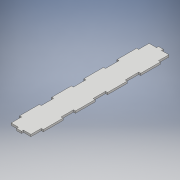
# Autodesk Inventor part: F3
Saved by Autodesk Inventor 2018 (Build 220112000, 112)
## iProperties
Created: 2018-03-06
Part Number: F3
Material: Generic
Document SubType Name: Modeling
Designer: isai
Density: 1 g/cm^3
Appearance: Default
Author: isai
Autodesk Inventor part; units mm, degrees
ref_plane "YZ Plane" through (0, 0, 0) normal (1, 0, 0) x (0, 1, 0)
ref_plane "XZ Plane" through (0, 0, 0) normal (0, 1, 0) x (-1, 0, 0)
ref_plane "XY Plane" through (0, 0, 0) normal (0, 0, 1) x (1, 0, 0)
sketch "Sketch1" plane through (0, 0, 0) normal (0, 0, 1) x (1, 0, 0)
  line L0 (29, -258.2) -> (29, -233.2)
  line L1 (29, -233.2) -> (25, -233.2)
  line L2 (25, -233.2) -> (25, -193.2)
  line L3 (25, -193.2) -> (29, -193.2)
  line L4 (29, -193.2) -> (29, -168.2)
  line L5 (29, -168.2) -> (25, -168.2)
  line L6 (25, -168.2) -> (25, -128.2)
  line L7 (25, -128.2) -> (29, -128.2)
  line L8 (29, -128.2) -> (29, -103.2)
  line L9 (29, -103.2) -> (25, -103.2)
  line L10 (25, -103.2) -> (25, -63.2)
  line L11 (25, -63.2) -> (29, -63.2)
  line L12 (29, -63.2) -> (29, -36)
  line L13 (29, -36) -> (25, -36)
  line L14 (25, -36) -> (25, 4)
  line L15 (25, 4) -> (29, 4)
  line L16 (29, 4) -> (29, 29)
  line L17 (29, 29) -> (29, 25)
  line L18 (29, 25) -> (69, 25)
  line L19 (29, -258.2) -> (29, -254.2)
  line L20 (29, -254.2) -> (69, -254.2)
  line L21 (49, 25) -> (49, 50.1757)
  line L22 (69, -63.2) -> (69, -36)
  line L23 (73, -36) -> (73, 4)
  line L24 (69, -36) -> (73, -36)
  line L25 (73, 4) -> (69, 4)
  line L26 (73, -233.2) -> (73, -193.2)
  line L27 (73, -193.2) -> (69, -193.2)
  line L28 (69, -233.2) -> (73, -233.2)
  line L29 (69, -168.2) -> (73, -168.2)
  line L30 (73, -168.2) -> (73, -128.2)
  line L31 (73, -63.2) -> (69, -63.2)
  line L32 (69, -103.2) -> (73, -103.2)
  line L33 (73, -128.2) -> (69, -128.2)
  line L34 (73, -103.2) -> (73, -63.2)
  line L35 (69, 25) -> (69, 4)
  line L36 (69, -36) -> (69, -63.2)
  line L37 (69, -103.2) -> (69, -128.2)
  line L38 (69, -168.2) -> (69, -193.2)
  line L39 (69, -233.2) -> (69, -254.2)
  point P0 (0, 0)
  dimension "d1" = 40
  dimension "d2" = 4
  dimension "d3" = 40
  dimension "d4" = 40
  dimension "d5" = 40
  dimension "d6" = 40
  dimension "d7" = 279.2
  constraints: 80 end point, 16 symmetric about line, 7 perpendicular, 2 point on line, 1 midpoint, 1 vertical
  measures "d1" distance of L17.end L18.end
  measures "d2" distance of L0.start L19.end
  measures "d3" distance of L2.start L2.end
  measures "d4" distance of L5.end L6.end
  measures "d5" distance of L9.end L11.start
  measures "d6" distance of L14.start L14.end
  measures "d7" distance of L18.end L20.end
extrude "Extrusion1" add sketch "Sketch1" along normal blind 4
sketch "Sketch2" plane through (0, 0, 4) normal (0, 0, 1) x (1, 0, 0)
  line L0 (25, -63.2) -> (25, -103.2) projected
  line L1 (25, -103.2) -> (29, -103.2) projected
  line L2 (29, -103.2) -> (29, -128.2) projected
  line L3 (29, -128.2) -> (25, -128.2) projected
  line L4 (25, -128.2) -> (25, -168.2) projected
  line L5 (25, -168.2) -> (29, -168.2) projected
  line L6 (29, -168.2) -> (29, -193.2) projected
  line L7 (29, -193.2) -> (25, -193.2) projected
  line L8 (25, -193.2) -> (25, -233.2) projected
  line L9 (25, -233.2) -> (29, -233.2) projected
  line L10 (29, -233.2) -> (29, -254.2) projected
  line L11 (29, -254.2) -> (69, -254.2) projected
  line L12 (69, -254.2) -> (69, -233.2) projected
  line L13 (69, -233.2) -> (73, -233.2) projected
  line L14 (73, -233.2) -> (73, -193.2) projected
  line L15 (73, -193.2) -> (69, -193.2) projected
  line L16 (69, -193.2) -> (69, -168.2) projected
  line L17 (69, -168.2) -> (73, -168.2) projected
  line L18 (73, -168.2) -> (73, -128.2) projected
  line L19 (73, -128.2) -> (69, -128.2) projected
  line L20 (69, -128.2) -> (69, -103.2) projected
  line L21 (69, -103.2) -> (73, -103.2) projected
  line L22 (73, -103.2) -> (73, -63.2) projected
  line L23 (73, -63.2) -> (69, -63.2) projected
  line L24 (69, -63.2) -> (69, -36) projected
  line L25 (69, -36) -> (73, -36) projected
  line L26 (73, -36) -> (73, 4) projected
  line L27 (73, 4) -> (69, 4) projected
  line L28 (69, 4) -> (69, 25) projected
  line L29 (69, 25) -> (29, 25) projected
  line L30 (29, 25) -> (29, 4) projected
  line L31 (29, 4) -> (25, 4) projected
  line L32 (25, 4) -> (25, -36) projected
  line L33 (25, -36) -> (29, -36) projected
  line L34 (29, -36) -> (29, -63.2) projected
  line L35 (29, -63.2) -> (25, -63.2) projected
  line L36 (44, 25) -> (54, 25)
  line L37 (54, 25) -> (54, 29)
  line L38 (54, 29) -> (44, 29)
  line L39 (44, 29) -> (44, 25)
  point P0 (0, 0)
  point P1 (49, 25)
  dimension "d10" = 10
  dimension "d11" = 4
  constraints: 8 end point, 2 midpoint, 2 parallel, 1 horizontal, 1 perpendicular
  measures "d10" distance of L38.end L37.end
  measures "d11" distance of L37.end L36.end
extrude "Extrusion2" add sketch "Sketch2" against normal blind 4 contours L39 L38 L37 L29
ref_plane "Work Plane1" through (29, -114.6, 0) normal (0, -1, 0) x (1, 0, 0)
mirror "Mirror1" about plane through (29, -114.6, 0) normal (0, -1, 0) of "Extrusion2"
equation "\"d3\" = D"
equation "\"d4\" = D"
equation "\"d5\" = D"
equation "\"d6\" = D"
equation "\"D\" = 40"
body "Solid1"
